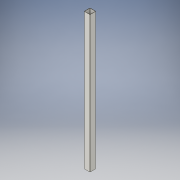
# Autodesk Inventor part: 3 x 3 TUBE .125 steel-69.75
Saved by Autodesk Inventor 2018.2 (Build 222227000, 227)
## iProperties
Created: 2017-12-18
Part Number: 3 x 3 TUBE .125 steel-69.75
Material: Steel
Document SubType Name: Modeling
Designer: torba
Density: 7.85 g/cm^3
Appearance: Steel
Author: torba
Autodesk Inventor part; units mm, degrees
ref_plane "YZ Plane" through (0, 0, 0) normal (1, 0, 0) x (0, 1, 0)
ref_plane "XZ Plane" through (0, 0, 0) normal (0, 1, 0) x (-1, 0, 0)
ref_plane "XY Plane" through (0, 0, 0) normal (0, 0, 1) x (1, 0, 0)
sketch "Sketch1" plane through (0, 0, 0) normal (0, 1, 0) x (-1, 0, 0)
  line L0 (0, 0) -> (76.2, 0)
  line L1 (76.2, 0) -> (76.2, -76.2)
  line L2 (76.2, -76.2) -> (0, -76.2)
  line L3 (0, -76.2) -> (0, 0)
  line L4 (73.025, -3.175) -> (3.175, -3.175)
  line L5 (3.175, -3.175) -> (3.175, -73.025)
  line L6 (3.175, -73.025) -> (73.025, -73.025)
  line L7 (73.025, -73.025) -> (73.025, -3.175)
  dimension "d0" = 76.2
  dimension "d1" = 76.2
  dimension "d2" = 3.175
  dimension "d3" = 3.175
  dimension "d4" = 3.175
  dimension "d5" = 3.175
  constraints: 16 end point, 4 parallel, 2 horizontal, 2 perpendicular
  measures "d0" distance between parallel lines of L2 L0
  measures "d1" distance between parallel lines of L3 L1
  measures "d2" distance between parallel lines of L1 L7
  measures "d3" distance between parallel lines of L2 L6
  measures "d4" distance between parallel lines of L3 L5
  measures "d5" distance between parallel lines of L0 L4
extrude "Extrusion1" add sketch "Sketch1" along normal blind 1771.65
fillet "Fillet1" radius 3.175 8 edges at (-73.025, 885.825, -73.025) (-76.2, 885.825, -76.2) (0, 885.825, -76.2) (-3.175, 885.825, -73.025) (0, 885.825, 0) (-3.175, 885.825, -3.175) (-76.2, 885.825, 0) (-73.025, 885.825, -3.175)
equation "\"d1\" = d0"
equation "\"d3\" = d2"
equation "\"d4\" = d2"
equation "\"d5\" = d2"
body "Solid1"
